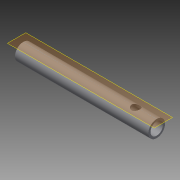
# Autodesk Inventor part: pin
Saved by Autodesk Inventor 2016 (Build 200138000, 138)
## iProperties
Created: 2015-10-13
Part Number: pin
Material: Generic
Document SubType Name: Modeling
Designer: eedoga
Density: 1 g/cm^3
Appearance: Default
Author: eedoga
Autodesk Inventor part; units mm, degrees
ref_plane "YZ Plane" through (0, 0, 0) normal (1, 0, 0) x (0, 1, 0)
ref_plane "XY Plane" through (0, 0, 0) normal (0, 0, 1) x (1, 0, 0)
sketch "Sketch1" plane through (0, 0, 0) normal (1, 0, 0) x (0, 1, 0)
  circle A0 centre (0, 0) radius 6.35
  circle A1 centre (0, 0) radius 4.7625
  dimension "d0" = 12.7
  constraints: 2 centre point, 2 coincident
  measures "d0" diameter of A0
extrude "Extrusion1" add sketch "Sketch1" along normal blind 101.6
ref_plane "Work Plane1" through (0, 6.35, 0) normal (0, 1, 0) x (-1, 0, 0)
sketch "Sketch2" plane through (0, 6.35, 0) normal (0, 1, 0) x (-1, 0, 0)
  line L0 (-101.6, 6.35) -> (-101.6, -6.35) projected
  line L1 (0, -6.35) -> (0, 6.35) projected
  line L2 (0, 0) -> (-101.6, 0)
  circle A0 centre (-85.725, 0) radius 3.81
  dimension "d3" = 7.62
  constraints: 2 end point, 1 centre point, 1 midpoint, 1 point on line
  measures "d3" diameter of A0
hole "Hole1" at (85.725, 6.35, 0) direction (0, -1, 0) diameter 6.35 end through all
body "Solid1"
